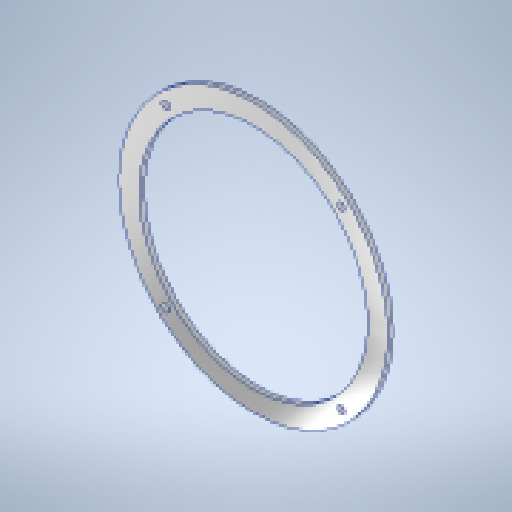
# Autodesk Inventor part: base_plate4
Saved by Autodesk Inventor 2024 (Build 280153000, 153)
## iProperties
Created: 2025-02-13
Part Number: base_plate4
Material: アルミニウム 6061
Document SubType Name: Modeling
Designer: tanoue_kota
Density: 2.7 g/cm^3
Appearance: アルミニウム - フラット
Author: tanoue_kota
Autodesk Inventor part; units mm, degrees
ref_plane "YZ Plane" through (0, 0, 0) normal (1, 0, 0) x (0, 1, 0)
ref_plane "XZ Plane" through (0, 0, 0) normal (0, 1, 0) x (-1, 0, 0)
ref_plane "XY Plane" through (0, 0, 0) normal (0, 0, 1) x (1, 0, 0)
sketch "スケッチ1" plane through (0, 0, 0) normal (0, 0, 1) x (1, 0, 0)
  circle A0 centre (0, 0) radius 42.25
  circle A1 centre (0, 0) radius 53.25
  circle A2 centre (0, 0) radius 49.25
  circle A3 centre (0, 0) radius 57.25
  dimension "d0" = 84.5
  dimension "d1" = 11
  dimension "d2" = 4
  dimension "d3" = 4
  constraints: 4 centre point, 4 coincident
  measures "d0" diameter of A0
  measures "d1" radial gap between concentric circles of A0 A1
  measures "d2" radial gap between concentric circles of A1 A2
  measures "d3" radial gap between concentric circles of A1 A3
extrude "押し出し1" add sketch "スケッチ1" along normal blind 2 contours A1 | A3
sketch "スケッチ2" plane through (0, 0, 2) normal (0, 0, 1) x (1, 0, 0)
  line L0 (0, 0) -> (0, 57.25)
  circle A0 centre (0, 0) radius 57.25 projected
  line L1 (0, 0) -> (40.4819, 40.4819)
  circle A1 centre (0, 0) radius 53.25
  circle A2 centre (0, 0) radius 49.25 projected
  point P0 (37.6534, 37.6534)
  point P1 (-37.6534, 37.6534)
  point P2 (-37.6534, -37.6534)
  point P3 (37.6534, -37.6534)
  dimension "d6" = 45
  dimension "d7" = 4
  dimension "d10" = 360
  constraints: 4 end point, 2 point on circle, 1 coincident, 1 point on line, 1 vertical, 8 other
  measures "d6" angle of L0 L1
hole "穴1" at (37.6534, 37.6534, 2) at (-37.6534, 37.6534, 2) at (-37.6534, -37.6534, 2) at (37.6534, -37.6534, 2) direction (0, 0, -1) diameter 3.1 end through all
